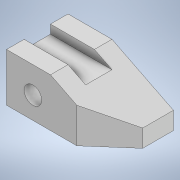
# Autodesk Inventor part: WedgeBlock
Saved by Autodesk Inventor 2022.2 (Build 262287030, 287C)
## iProperties
Created: 2023-02-22
Part Number: WedgeBlock
Material: Generic
Document SubType Name: Modeling
Designer: jak27277
Density: 1 g/cm^3
Appearance: Default
Mass: 650.55 g
Surface Area: 583.698 cm^2
Volume: 650.55 cm^3
Author: jak27277
Autodesk Inventor part; units mm, degrees
ref_plane "YZ Plane" through (0, 0, 0) normal (1, 0, 0) x (0, 1, 0)
ref_plane "XZ Plane" through (0, 0, 0) normal (0, 1, 0) x (-1, 0, 0)
ref_plane "XY Plane" through (0, 0, 0) normal (0, 0, 1) x (1, 0, 0)
sketch "Sketch1" plane through (0, 0, 0) normal (1, 0, 0) x (0, 1, 0)
  line L0 (0, 0) -> (69.85, 0)
  line L1 (69.85, 0) -> (69.85, -88.9)
  line L2 (69.85, -88.9) -> (0, -88.9)
  line L3 (0, -88.9) -> (0, 0)
  dimension "d0" = 88.9
  dimension "d1" = 69.85
  constraints: 8 end point, 2 parallel, 1 horizontal, 1 perpendicular
  measures "d0" distance of L0.end L1.end
  measures "d1" distance of L0.start L0.end
extrude "Extrusion1" add sketch "Sketch1" along normal blind 152.4
sketch "Sketch4" plane through (152.4, 0, 0) normal (1, 0, 0) x (0, 0, -1)
  line L0 (88.9, 69.85) -> (0, 69.85) projected
  line L1 (25.4, 69.85) -> (63.5, 69.85)
  line L2 (63.5, 69.85) -> (63.5, 57.15)
  line L3 (63.5, 57.15) -> (25.4, 57.15)
  line L4 (25.4, 57.15) -> (25.4, 69.85)
  line L5 (88.9, 0) -> (88.9, 69.85) projected
  point P0 (0, 0)
  point P1 (63.5, 69.85)
  dimension "d6" = 38.1
  dimension "d7" = 25.4
  dimension "d8" = 12.7
  constraints: 8 end point, 2 parallel, 1 horizontal, 1 perpendicular, 1 point on line
  measures "d6" distance of L2.end L3.end
  measures "d7" distance between parallel lines of L5 L2
  measures "d8" distance of L3.end L1.start
extrude "Extrusion3" cut sketch "Sketch4" against normal through all
sketch "Sketch5" plane through (0, 0, 0) normal (0, 0, 1) x (1, 0, 0)
  line L0 (0, 69.85) -> (152.4, 69.85) projected
  line L1 (63.5, 69.85) -> (152.4, 25.4)
  line L2 (152.4, 69.85) -> (152.4, 0) projected
  line L3 (0, 69.85) -> (0, 0) projected
  line L4 (0, 0) -> (152.4, 0) projected
  line L5 (152.4, 69.85) -> (152.4, 0) projected
  line L6 (0, 69.85) -> (152.4, 69.85) projected
  dimension "d28" = 25.4
  dimension "d29" = 63.5
  constraints: 2 end point, 2 point on line
  measures "d28" distance of L2.end L1.end
  measures "d29" distance from line of L3 L1.start
extrude "Extrusion4" cut sketch "Sketch5" against normal through all contours L0 L2 L1
sketch "Sketch6" plane through (0, 69.85, -63.5) normal (0, 1, 0) x (1, 0, 0)
  line L0 (152.4, 25.4) -> (152.4, -63.5) projected
  line L1 (152.4, -19.05) -> (101.6, -63.5)
  line L2 (0, -63.5) -> (152.4, -63.5) projected
  line L3 (0, 25.4) -> (0, -63.5) projected
  line L4 (0, 25.4) -> (0, -63.5) projected
  line L5 (0, 25.4) -> (152.4, 25.4) projected
  line L6 (63.5, 25.4) -> (152.4, 25.4) projected
  point P0 (0, -38.1)
  point P1 (0, 0)
  dimension "d22" = 101.6
  dimension "d30" = 44.45
  constraints: 2 end point, 1 midpoint, 1 point on line
  measures "d22" distance from line of L3 L1.end
  measures "d30" distance from line of L1.start L6
extrude "Extrusion5" cut sketch "Sketch6" against normal through all contours L0 L2 L1
sketch "Sketch8" plane through (0, 0, 0) normal (0, 0, 1) x (1, 0, 0)
  line L0 (0, 69.85) -> (0, 0) projected
  line L1 (0, 0) -> (101.6, 0) projected
  point P0 (38.1, 31.75)
  dimension "d31" = 38.1
  dimension "d32" = 31.75
  measures "d31" distance from line of point (38.1, 31.75) L0
  measures "d32" distance from line of L1 point (38.1, 31.75)
hole "Hole1" at (38.1, 31.75, 0) direction (0, 0, -1) diameter 25.4 end through all
body "Solid1"
